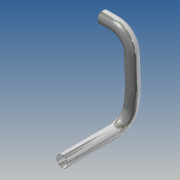
# Autodesk Inventor part: exhaust header right pipe 6
Saved by Autodesk Inventor 2013 (Build 170138000, 138)
## iProperties
Created: 2013-02-09
Part Number: exhaust header right pipe 6
Material: Steel
Document SubType Name: Modeling
Designer: zhaphod
Density: 1 g/cm^3
Author: zhaphod
Autodesk Inventor part; units mm, degrees
sketch "Sketch1" plane through (0, 0, 0) normal (1, 0, 0) x (0, 1, 0)
  line L0 (0, 0) -> (0, -175)
  line L1 (0, -175) -> (0, -287.775)
  line L2 (0, -287.775) -> (-247.4, -287.775)
  line L3 (0, 0) -> (0, -103.1875) construction
  line L4 (0, -103.1875) -> (0, -109.925) construction
  line L5 (0, -109.925) -> (0, -97.225) construction
  line L6 (0, -97.225) -> (-247.4, -97.225) construction
  dimension "d0" = 287.775
  dimension "d1" = 0
  dimension "d4" = 175
  dimension "d5" = 247.4
  dimension "d6" = 103.1875
  dimension "d7" = 97.225
  dimension "d8" = 109.925
  constraints: 14 end point, 3 vertical alignment, 2 perpendicular, 1 horizontal, 1 vertical
  measures "d0" distance from line of L2 L0.start
  measures "d1" horizontal distance of L0.end L0.start
  measures "d4" distance of L0.end L0.start
  measures "d5" horizontal distance of L0.start L2.end
  measures "d6" distance of L0.start L3.end
  measures "d7" distance from line of L6 L0.start
  measures "d8" distance of L4.end L0.start
ref_plane "Work Plane1" through (103.1875, 0, 0) normal (1, 0, 0) x (0, 1, 0)
ref_plane "Work Plane2" through (109.925, 0, 0) normal (1, 0, 0) x (0, 1, 0)
ref_plane "Work Plane3" through (97.225, 0, 0) normal (1, 0, 0) x (0, 1, 0)
sketch "Sketch2" plane through (103.1875, 0, 0) normal (1, 0, 0) x (0, 1, 0)
  point P0 (0, 0)
  point P1 (0, 0)
sketch "Sketch3" plane through (109.925, 0, 0) normal (1, 0, 0) x (0, 1, 0)
  point P0 (0, 0)
  point P1 (0, -175)
  point P2 (0, -287.775)
sketch "Sketch4" plane through (97.225, 0, 0) normal (1, 0, 0) x (0, 1, 0)
  point P0 (0, 0)
  point P1 (-247.4, -287.775)
  point P2 (0, -287.775)
sketch "Sketch5" plane through (0, 0, 0) normal (1, 0, 0) x (0, 1, 0)
  circle A0 centre (0, 0) radius 20.6375
  circle A1 centre (0, 0) radius 19.0375
  dimension "d15" = 1.6
  dimension "d17" = 41.275
  constraints: 2 centre point, 2 coincident
  measures "d15" radial gap between concentric circles of A0 A1
  measures "d17" diameter of A0
sketch3d "3D Sketch1"
  line L0 (0, 0, 0) -> (43.6128, 0, 0)
  arc A0 (43.6128, 0, 0) -> (105.4794, 0, -59.5306) centre (43.6128, 0, -61.9125) ccw
  line L1 (105.4794, 0, -59.5306) -> (109.7453, 0, -170.3319)
  arc A1 (109.7453, 0, -170.3319) -> (109.4022, 0, -179.6422) centre (47.8786, 0, -172.7138) ccw
  line L2 (109.4022, 0, -179.6422) -> (104.1534, 0, -226.2514)
  arc A2 (104.1534, 0, -226.2514) -> (97.225, -61.9125, -287.775) centre (104.1534, -61.9125, -226.2514) ccw
  line L3 (97.225, -61.9125, -287.775) -> (97.225, -247.4, -287.775)
  dimension "d14" = 61.9125
  dimension "d12" = 61.9125
  dimension "d13" = 61.9125
  constraints: 4 vertical
sweep "Sweep1" add profiles "Sketch5" path "3D Sketch1"
equation "\"d14\" = d12"
equation "\"d13\" = d12"
equation "\"d9\" = d6"
equation "\"d10\" = d8"
equation "\"d11\" = d7"
body "Solid1"
